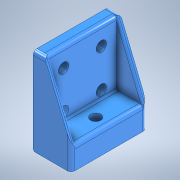
# Autodesk Inventor part: Foot_Bracket
Saved by Autodesk Inventor 2021 (Build 250183000, 183)
## iProperties
Created: 2021-05-18
Part Number: Foot_Bracket
Material: Generic
Document SubType Name: Modeling
Designer: Jorian Brusind
Density: 1 g/cm^3
Appearance: Cyan
Author: Jorian Brusind
Autodesk Inventor part; units mm, degrees
ref_plane "YZ Plane" through (0, 0, 0) normal (1, 0, 0) x (0, 1, 0)
ref_plane "XZ Plane" through (0, 0, 0) normal (0, 1, 0) x (-1, 0, 0)
ref_plane "XY Plane" through (0, 0, 0) normal (0, 0, 1) x (1, 0, 0)
sketch "Sketch1" plane through (0, 0, 0) normal (0, 1, 0) x (-1, 0, 0)
  line L0 (0, 0) -> (20, 0)
  line L1 (20, 0) -> (20, -40)
  line L2 (20, -40) -> (0, -40)
  line L3 (0, -40) -> (0, 0)
  dimension "d0" = 20
  dimension "d1" = 40
  constraints: 8 end point, 2 parallel, 1 horizontal, 1 perpendicular
  measures "d0" distance of L1.end L2.end
  measures "d1" distance of L0.end L1.end
extrude "Extrusion1" add sketch "Sketch1" along normal blind 12
sketch "Sketch2" plane through (0, 12, 0) normal (0, 1, 0) x (1, 0, 0)
  line L0 (-20, 40) -> (-20, 0) projected
  line L1 (-20, 0) -> (-14, 0)
  line L2 (-14, 0) -> (-14, 40)
  line L3 (-14, 40) -> (-20, 40)
  line L4 (-20, 40) -> (-20, 0)
  point P0 (0, 0)
  dimension "d4" = 6
  dimension "d5" = 40
  constraints: 8 end point, 2 parallel, 1 horizontal, 1 perpendicular
  measures "d4" distance of L3.end L2.end
  measures "d5" distance of L2.end L1.end
extrude "Extrusion2" add sketch "Sketch2" along normal blind 34
sketch "Sketch3" plane through (0, 0, 0) normal (0, -1, 0) x (1, 0, 0)
  circle A0 centre (-7, -20) radius 2.75
  line L0 (0, 0) -> (0, -40) projected
  line L1 (-20, 0) -> (0, 0) projected
  dimension "d8" = 5.5
  dimension "d9" = 7
  dimension "d10" = 20
  constraints: 1 centre point
  measures "d8" diameter of A0
  measures "d9" distance from line of L0 A0.centre
  measures "d10" distance from line of L1 A0.centre
extrude "Extrusion3" cut sketch "Sketch3" against normal through all
sketch "Sketch4" plane through (0, 0, 0) normal (0, -1, 0) x (1, 0, 0)
  circle A0 centre (-7, -20) radius 2.75 projected
  line L0 (-2.3812, -20) -> (-4.6906, -24)
  line L1 (-4.6906, -24) -> (-9.3094, -24)
  line L2 (-9.3094, -24) -> (-11.6188, -20)
  line L3 (-11.6188, -20) -> (-9.3094, -16)
  line L4 (-9.3094, -16) -> (-4.6906, -16)
  line L5 (-4.6906, -16) -> (-2.3812, -20)
  line L6 (-14, -40) -> (-14, 0) projected
  point P0 (0, 0)
  dimension "d13" = 8
  dimension "d14" = 90
  constraints: 12 end point, 1 coincident, 13 other
  measures "d13" distance between parallel lines of L1 L4
  measures "d14" angle of L6 L1
extrude "Extrusion4" cut sketch "Sketch4" against normal blind 4
sketch "Sketch5" plane through (0, 0, 0) normal (0, -1, 0) x (1, 0, 0)
  circle A0 centre (-4, -5) radius 2.75
  line L0 (0, 0) -> (0, -40) projected
  line L1 (-20, 0) -> (0, 0) projected
  circle A1 centre (-4, -35) radius 2.75
  circle A2 centre (-16, -5) radius 2.75
  circle A3 centre (-16, -35) radius 2.75
  dimension "d17" = 5.5
  dimension "d18" = 4
  dimension "d19" = 5
  dimension "d22" = 30
  dimension "d25" = 12
  constraints: 4 centre point, 1 horizontal, 1 vertical, 6 other
  measures "d17" diameter of A0
  measures "d18" distance from line of L0 A0.centre
  measures "d19" distance from line of L1 A0.centre
  measures "d22" distance of A0.centre A1.centre
  measures "d25" distance of A0.centre A2.centre
extrude "Extrusion5" cut sketch "Sketch5" against normal blind 8
sketch "Sketch6" plane through (-14, 12, 0) normal (1, 0, 0) x (0, 0, -1)
  circle A0 centre (10, 24) radius 2.75
  line L0 (0, 34) -> (40, 34) projected
  line L1 (0, 0) -> (0, 34) projected
  circle A1 centre (10, 4) radius 2.75
  point P0 (0, -12)
  dimension "d30" = 5.5
  dimension "d31" = 10
  dimension "d32" = 10
  dimension "d33" = 5.5
  dimension "d34" = 20
  dimension "d35" = 10
  constraints: 2 centre point
  measures "d30" diameter of A0
  measures "d31" distance from line of L0 A0.centre
  measures "d32" distance from line of L1 A0.centre
  measures "d33" diameter of A1
  measures "d34" distance of A0.centre A1.centre
  measures "d35" distance from line of L1 A1.centre
extrude "Extrusion6" cut sketch "Sketch6" against normal through all
sketch "Sketch7" plane through (-20, 0, 0) normal (0, 0, 1) x (1, 0, 0)
  line L0 (6, 12) -> (6, 46) projected
  line L1 (6, 46) -> (6, 12)
  line L2 (20, 12) -> (6, 12) projected
  line L3 (6, 12) -> (20, 12)
  line L4 (20, 12) -> (6, 46)
  point P0 (20, 0)
  point P1 (0, 6)
  constraints: 6 end point, 1 collinear, 1 horizontal, 1 other
extrude "Extrusion7" add sketch "Sketch7" against normal blind 2
pattern_linear "Rectangular Pattern1" count 2 spacing 38 along (0, 0, -1) of "Extrusion7"
fillet "Fillet1" radius 2 2 edges at (-14, 46, -20) (0, 12, -20)
fillet "Fillet2" radius 2 2 edges at (0, 6, 0) (0, 6, -40)
fillet "Fillet3" radius 2 2 edges at (-17, 46, 0) (-17, 46, -40)
fillet "Fillet4" radius 1 2 edges at (-7, 29, -2) (-7, 29, -38)
fillet "Fillet5" radius 1 1 edges at (-20, 0, -20)
sketch "Sketch8" plane through (-14, 12, -2) normal (1, 0, 0) x (0, 0, -1)
  circle A0 centre (28, 24) radius 2.75
  circle A1 centre (8, 24) radius 2.75 projected
  line L0 (-0.0289, 32) -> (36.0289, 32) projected
  circle A2 centre (28, 4) radius 2.75
  circle A3 centre (8, 4) radius 2.75 projected
  point P0 (-2, -12)
  dimension "d48" = 5.5
  dimension "d49" = 20
  dimension "d50" = 8
  dimension "d51" = 5.5
  dimension "d52" = 20
  dimension "d53" = 20
  constraints: 2 centre point
  measures "d48" diameter of A0
  measures "d49" distance of A1.centre A0.centre
  measures "d50" distance from line of L0 A0.centre
  measures "d51" diameter of A2
  measures "d52" distance of A2.centre A0.centre
  measures "d53" distance of A3.centre A2.centre
extrude "Extrusion8" cut sketch "Sketch8" against normal through all contours A0 | A2
fillet "Fillet6" radius 1 1 edges at (-14, 12, -20)
body "Solid1"
